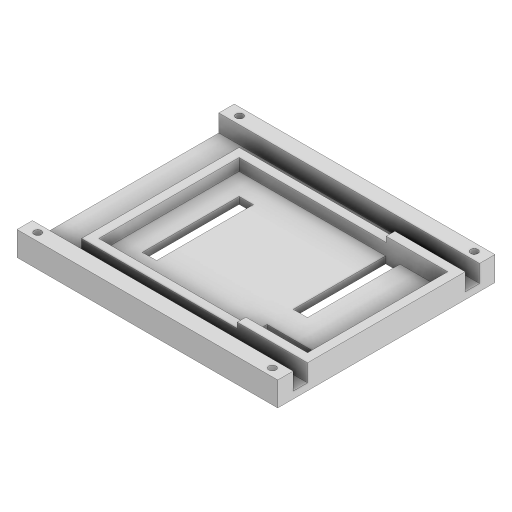
# Autodesk Inventor part: RFID_Bottom
Saved by Autodesk Inventor 2023 (Build 270158000, 158)
## iProperties
Created: 2022-10-13
Part Number: RFID_Bottom
Material: Generic
Document SubType Name: Modeling
Designer: Vking
Density: 1 g/cm^3
Appearance: Default
Author: Vking
Autodesk Inventor part; units mm, degrees
ref_plane "YZ Plane" through (0, 0, 0) normal (1, 0, 0) x (0, 1, 0)
ref_plane "XZ Plane" through (0, 0, 0) normal (0, 1, 0) x (-1, 0, 0)
ref_plane "XY Plane" through (0, 0, 0) normal (0, 0, 1) x (1, 0, 0)
sketch "Sketch1" plane through (0, 0, 0) normal (0, 1, 0) x (-1, 0, 0)
  line L0 (31, 20.5) -> (-30, 20.5)
  line L1 (-30, 20.5) -> (-30, -20.5)
  line L2 (-30, -20.5) -> (31, -20.5)
  line L3 (31, -20.5) -> (31, 20.5)
  line L4 (33.54, 23.04) -> (-32.54, 23.04)
  line L5 (-32.54, 23.04) -> (-32.54, -23.04)
  line L6 (-32.54, -23.04) -> (33.54, -23.04)
  line L7 (33.54, -23.04) -> (33.54, 23.04)
  line L8 (-12, -20.5) -> (-12, 20.5)
  line L9 (-12, -23.04) -> (-12, -20.5)
  line L10 (-12, 20.5) -> (-12, 23.04)
  point P0 (0, 0)
  dimension "d0" = 41
  dimension "d1" = 61
  dimension "d2" = 20.5
  dimension "d3" = 31
  dimension "d4" = 2.54
  dimension "d9" = 18
  dimension "d48" = 46.08
  constraints: 22 end point, 5 point on line, 4 parallel, 3 perpendicular, 1 horizontal, 1 vertical, 3 other
  measures "d0" distance of L2.end L0.start
  measures "d1" distance of L1.end L2.end
  measures "d2" distance from line of point (0, 0) L2
  measures "d3" distance from line of point (0, 0) L3
  measures "d4" distance between parallel lines of L3 L7
  measures "d9" distance between parallel lines of L1 L8
  measures "d48" distance of L6.end L4.start
extrude "Extrusion1" add sketch "Sketch1" along normal blind 3.5 contours L0 L10 L4 L7 L6 L9 L2 L3
extrude "Extrusion3" add sketch "Sketch1" along normal blind 5.08 contours L0 L1 L2 L9 L6 L5 L4 L10
sketch "Sketch3" plane through (0, 0, 0) normal (0, -1, 0) x (1, 0, 0)
  line L0 (-31, -20.5) -> (30, -20.5) projected
  line L1 (-31, 20.5) -> (-31, -20.5) projected
  line L2 (30, 20.5) -> (-31, 20.5) projected
  line L3 (30, -20.5) -> (30, 20.5) projected
  line L4 (32.54, -23.04) -> (-33.54, -23.04) projected
  line L5 (32.54, 23.04) -> (32.54, -23.04) projected
  line L6 (-33.54, 23.04) -> (32.54, 23.04) projected
  line L7 (-33.54, -23.04) -> (-33.54, 23.04) projected
  point P0 (0, 0)
extrude "Extrusion4" add sketch "Sketch3" along normal blind 1 contours L1 L2 L3 L0 | L4 L7 L6 L5
sketch "Sketch4" plane through (0, 0, 0) normal (0, 1, 0) x (1, 0, 0)
  line L0 (12, -20.5) -> (-31, -20.5) projected
  line L1 (-31, -20.5) -> (-31, 20.5) projected
  line L2 (30, 20.5) -> (30, -20.5) projected
  line L3 (30, -20.5) -> (12, -20.5) projected
  line L4 (-31, 20.5) -> (12, 20.5) projected
  line L5 (-24.65, 20.5) -> (-20.459, 20.5)
  line L6 (-20.459, 20.5) -> (-20.459, -20.5)
  line L7 (-20.459, -20.5) -> (-24.65, -20.5)
  line L8 (-24.65, -20.5) -> (-24.65, 20.5)
  line L9 (16.03, -20.5) -> (11.839, -20.5)
  line L10 (11.839, -20.5) -> (11.839, 20.5)
  line L11 (11.839, 20.5) -> (16.03, 20.5)
  line L12 (16.03, 20.5) -> (16.03, -20.5)
  point P0 (0, 0)
  point P1 (-24.65, -20.5)
  dimension "d31" = 4.191
  dimension "d37" = 4.191
  dimension "d38" = 13.97
  dimension "d45" = 6.35
  constraints: 16 end point, 4 parallel, 4 point on line, 2 horizontal, 2 perpendicular
  measures "d31" distance between parallel lines of L10 L12
  measures "d37" distance between parallel lines of L8 L6
  measures "d38" distance between parallel lines of L2 L12
  measures "d45" distance between parallel lines of L1 L8
extrude "Extrusion5" cut sketch "Sketch4" against normal blind 25.4 contours L0 L10 L4 L11 L12 L3 | L0 L8 L4 L6
sketch "Sketch6" plane through (0, 0, 0) normal (0, 1, 0) x (1, 0, 0)
  line L0 (30, 20.5) -> (-31, 20.5) projected
  line L1 (30, -20.5) -> (16.03, -20.5) projected
  line L2 (30, 20.5) -> (27, 20.5)
  line L3 (27, 20.5) -> (27, -20.5)
  line L4 (27, -20.5) -> (30, -20.5)
  line L5 (30, -20.5) -> (30, 20.5)
  point P0 (0, 0)
  dimension "d33" = 3
  constraints: 8 end point, 2 parallel, 1 horizontal, 1 perpendicular, 1 point on line
  measures "d33" distance between parallel lines of L5 L3
extrude "Extrusion7" cut sketch "Sketch6" against normal blind 25.4
sketch "Sketch7" plane through (0, 0, 0) normal (0, 1, 0) x (1, 0, 0)
  line L0 (11.839, -20.5) -> (16.03, -20.5) projected
  line L1 (27, -20.5) -> (27, 20.5) projected
  line L2 (16.03, -20.5) -> (27, -20.5)
  line L3 (27, -20.5) -> (27, -16.69)
  line L4 (27, -16.69) -> (16.03, -16.69)
  line L5 (16.03, -16.69) -> (16.03, -20.5)
  line L6 (27, -20.5) -> (16.03, -20.5) projected
  line L7 (19.6495, -16.69) -> (22.1895, -16.69)
  line L8 (22.1895, -20.5) -> (19.6495, -20.5)
  point P0 (0, 0)
  dimension "d39" = 3.81
  dimension "d41" = 10.97
  constraints: 12 end point, 3 parallel, 3 point on line, 2 horizontal, 1 perpendicular
  measures "d39" distance between parallel lines of L2 L4
  measures "d41" distance of L3.end L4.end
extrude "Extrusion8" cut sketch "Sketch7" against normal blind 25.4
sketch "Sketch9" plane through (0, -1, 0) normal (0, -1, 0) x (1, 0, 0)
  line L0 (32.54, 31.7522) -> (-43.66, 31.7522)
  line L1 (-43.66, 31.7522) -> (-43.66, -31.7478)
  line L2 (-43.66, -31.7478) -> (32.54, -31.7478)
  line L3 (32.54, -31.7478) -> (32.54, 31.7522)
  line L4 (32.54, -23.04) -> (32.54, 23.04) projected
  line L5 (-33.54, 23.04) -> (-33.54, -23.04) projected
  line L6 (27, 16.69) -> (16.03, 16.69) projected
  line L7 (16.03, 16.69) -> (16.03, -20.5) projected
  line L8 (16.03, -20.5) -> (11.839, -20.5) projected
  line L9 (11.839, -20.5) -> (11.839, 20.5) projected
  line L10 (11.839, 20.5) -> (30, 20.5) projected
  line L11 (30, 20.5) -> (30, -20.5) projected
  line L12 (30, -20.5) -> (27, -20.5) projected
  line L13 (27, -20.5) -> (27, 16.69) projected
  line L14 (-20.459, 20.5) -> (-20.459, -20.5) projected
  line L15 (-20.459, -20.5) -> (-24.65, -20.5) projected
  line L16 (-24.65, -20.5) -> (-24.65, 20.5) projected
  line L17 (-24.65, 20.5) -> (-20.459, 20.5) projected
  line L18 (32.54, 23.04) -> (-33.54, 23.04) projected
  line L19 (-33.54, 23.04) -> (-33.54, -23.04) projected
  line L20 (-33.54, -23.04) -> (32.54, -23.04) projected
  line L21 (32.54, -23.04) -> (32.54, 23.04) projected
  point P0 (0, 0)
  point P1 (-33.54, -23.04)
  dimension "d46" = 0
  dimension "d49" = 8.7122
  dimension "d50" = 63.5
  dimension "d51" = 8.7078
  dimension "d52" = 76.2
  constraints: 8 end point, 2 parallel, 1 horizontal, 1 perpendicular
  measures "d46" distance between parallel lines of L4 L3
  measures "d49" distance between parallel lines of L0 L18
  measures "d50" distance of L2.end L0.start
  measures "d51" distance between parallel lines of L20 L2
  measures "d52" distance of L1.end L2.end
extrude "Extrusion9" add sketch "Sketch9" against normal blind 1 contours L3 L18 L5 L20 L2 L1 L0
sketch "Sketch10" plane through (0, 0, 0) normal (0, 1, 0) x (1, 0, 0)
  circle A0 centre (-39.85, 29.4978) radius 1.05
  line L0 (-43.66, 31.7478) -> (-43.66, 27.2478)
  circle A1 centre (-39.85, -29.5022) radius 1.05
  line L1 (-43.66, -27.2522) -> (-43.66, -31.7522)
  circle A2 centre (28.73, 29.4978) radius 1.05
  line L2 (32.54, 27.2478) -> (32.54, 31.7478)
  line L3 (-43.66, 27.2478) -> (32.54, 27.2478)
  circle A3 centre (28.73, -29.5022) radius 1.05
  line L4 (-43.66, -31.7522) -> (32.54, -31.7522)
  line L5 (32.54, -31.7522) -> (32.54, -27.2522)
  line L6 (-43.66, 31.7478) -> (-43.66, -31.7522)
  line L7 (-43.66, -31.7522) -> (32.54, -31.7522)
  line L8 (32.54, 31.7478) -> (32.54, -31.7522)
  line L9 (-43.66, 31.7478) -> (32.54, 31.7478)
  line L10 (-43.66, 31.7478) -> (-43.66, -31.7522) projected
  line L11 (-43.66, -31.7522) -> (32.54, -31.7522) projected
  line L12 (32.54, -31.7522) -> (-43.66, -31.7522)
  line L13 (-43.66, -31.7522) -> (-43.66, -27.2522)
  line L14 (-43.66, -27.2522) -> (32.54, -27.2522)
  line L15 (32.54, -27.2522) -> (32.54, -31.7522)
  point P0 (32.54, -0.0022)
  dimension "d55" = 2.1
  dimension "d56" = 3.81
  dimension "d57" = 2.25
  dimension "d58" = 2.25
  dimension "d59" = 2.1
  dimension "d60" = 3.81
  dimension "d61" = 2.1
  dimension "d62" = 2.1
  dimension "d63" = 3.81
  dimension "d64" = 3.81
  dimension "d65" = 2.25
  dimension "d66" = 2.25
  dimension "d67" = 4.5
  dimension "d68" = 4.5
  constraints: 28 end point, 4 centre point, 2 parallel, 1 coincident, 1 horizontal, 1 perpendicular, 1 point on line
  measures "d55" diameter of A2
  measures "d56" distance from line of L2 A2.centre
  measures "d57" distance from line of A2.centre L3
  measures "d58" distance from line of L4 A3.centre
  measures "d59" diameter of A3
  measures "d60" distance from line of L5 A3.centre
  measures "d61" diameter of A1
  measures "d62" diameter of A0
  measures "d63" distance from line of A1.centre L1
  measures "d64" distance from line of A0.centre L0
  measures "d65" distance from line of L3 A0.centre
  measures "d66" distance from line of L4 A1.centre
  measures "d67" distance between parallel lines of L9 L3
  measures "d68" distance between parallel lines of L11 L14
extrude "Extrusion10" add sketch "Sketch10" along normal blind 5.08 contours L9 L2 L3 L0 | L14 L5 L4 L1
sketch "Sketch11" plane through (0, 5.08, 0) normal (0, 1, 0) x (1, 0, 0)
  line L0 (-43.66, 31.7478) -> (-43.66, 27.2478) projected
  line L1 (-43.66, 27.2478) -> (32.54, 27.2478) projected
  line L2 (32.54, 27.2478) -> (32.54, 31.7478) projected
  line L3 (32.54, 31.7478) -> (-43.66, 31.7478) projected
  circle A0 centre (-39.85, 29.4978) radius 1.05 projected
  circle A1 centre (28.73, 29.4978) radius 1.05 projected
  line L4 (-43.66, -27.2522) -> (-43.66, -31.7522) projected
  line L5 (-43.66, -31.7522) -> (32.54, -31.7522) projected
  line L6 (32.54, -31.7522) -> (32.54, -27.2522) projected
  line L7 (32.54, -27.2522) -> (-43.66, -27.2522) projected
  circle A2 centre (28.73, -29.5022) radius 1.05 projected
  circle A3 centre (-39.85, -29.5022) radius 1.05 projected
  point P0 (0, 0)
extrude "Extrusion11" cut sketch "Sketch11" against normal blind 25.4 contours A0 | A1 | A2 | A3
sketch "Sketch12" plane through (0, 0, 0) normal (0, 1, 0) x (1, 0, 0)
  line L0 (16.03, -16.69) -> (16.03, 20.5) projected
  line L1 (27, 20.5) -> (27, -16.69) projected
  line L2 (16.03, -16.69) -> (27, -16.69)
  line L3 (27, -16.69) -> (27, -14.15)
  line L4 (27, -14.15) -> (16.03, -14.15)
  line L5 (16.03, -14.15) -> (16.03, -16.69)
  line L6 (11.839, 20.5) -> (11.839, -20.5) projected
  line L7 (11.839, -14.15) -> (16.03, -14.15)
  line L8 (16.03, -14.15) -> (16.03, -6.53)
  line L9 (16.03, -6.53) -> (11.839, -6.53)
  line L10 (11.839, -6.53) -> (11.839, -14.15)
  line L11 (30, -20.5) -> (12, -20.5) projected
  line L12 (-24.65, -20.5) -> (-24.65, 20.5) projected
  line L13 (-20.459, -20.5) -> (-20.459, 20.5) projected
  line L14 (-24.65, -20.5) -> (-20.459, -20.5)
  line L15 (-20.459, -20.5) -> (-20.459, -14.15)
  line L16 (-20.459, -14.15) -> (-24.65, -14.15)
  line L17 (-24.65, -14.15) -> (-24.65, -20.5)
  line L18 (-24.65, 20.5) -> (-20.459, 20.5)
  line L19 (-20.459, 20.5) -> (-20.459, 14.15)
  line L20 (-20.459, 14.15) -> (-24.65, 14.15)
  line L21 (-24.65, 14.15) -> (-24.65, 20.5)
  point P0 (0, 0)
  point P1 (27, -16.69)
  point P2 (11.839, -6.53)
  point P3 (21, -20.5)
  point P4 (13.9345, -14.15)
  dimension "d78" = 2.54
  dimension "d79" = 0
  dimension "d80" = 7.62
  dimension "d81" = 6.35
  dimension "d82" = 6.35
  constraints: 32 end point, 8 parallel, 5 point on line, 4 horizontal, 4 perpendicular, 2 midpoint
  measures "d78" distance between parallel lines of L2 L4
  measures "d79" vertical distance of L4.end point (13.934, -14.15)
  measures "d80" distance between parallel lines of L7 L9
  measures "d81" distance between parallel lines of L18 L20
  measures "d82" distance between parallel lines of L14 L16
extrude "Extrusion12" cut sketch "Sketch12" against normal blind 25.4 contours L0 L4 L1 L2
extrude "Extrusion13" add sketch "Sketch12" against normal blind 1 contours L7 L6 L9 L0 | L12 L16 L13 L14 | L12 L18 L13 L20
sketch "Sketch13" plane through (0, -1, 0) normal (0, -1, 0) x (1, 0, 0)
  line L0 (11.839, 20.5) -> (-31, 20.5) projected
  line L1 (16.03, 6.53) -> (16.03, -20.5) projected
  line L2 (16.03, -20.5) -> (11.839, -20.5) projected
  line L3 (11.839, -20.5) -> (11.839, 6.53) projected
  line L4 (11.839, 6.53) -> (16.03, 6.53) projected
  line L5 (32.54, -31.7478) -> (32.54, 31.7522) projected
  line L6 (32.54, 31.7522) -> (-43.66, 31.7522) projected
  line L7 (-43.66, 31.7522) -> (-43.66, -31.7478) projected
  line L8 (-43.66, -31.7478) -> (32.54, -31.7478) projected
  line L9 (-20.459, 14.15) -> (-20.459, -14.15) projected
  line L10 (-20.459, -14.15) -> (-24.65, -14.15) projected
  line L11 (-24.65, -14.15) -> (-24.65, 14.15) projected
  line L12 (-24.65, 14.15) -> (-20.459, 14.15) projected
  line L13 (27, 14.15) -> (11.839, 14.15) projected
  line L14 (11.839, 14.15) -> (11.839, 20.5) projected
  line L15 (11.839, 20.5) -> (30, 20.5) projected
  line L16 (30, 20.5) -> (30, -20.5) projected
  line L17 (30, -20.5) -> (27, -20.5) projected
  line L18 (27, -20.5) -> (27, 14.15) projected
  circle A0 centre (28.73, 29.5022) radius 1.05 projected
  circle A1 centre (28.73, -29.4978) radius 1.05 projected
  circle A2 centre (-39.85, 29.5022) radius 1.05 projected
  circle A3 centre (-39.85, -29.4978) radius 1.05 projected
  point P0 (0, 0)
extrude "Extrusion14" add sketch "Sketch13" along normal blind 1
body "Solid1"
